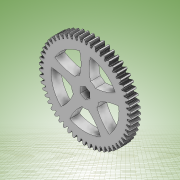
# Autodesk Inventor part: Engranaje1
Saved by Autodesk Inventor 2022 (Build 260153000, 153)
## iProperties
Created: 2022-03-08
Part Number: Engranaje1
Material: Genérico
Document SubType Name: Modeling
Designer: Marco
Density: 1 g/cm^3
Appearance: Valor por defecto
Author: Marco
Autodesk Inventor part; units mm, degrees
(part 1 of 3)
ref_plane "YZ Plane" through (0, 0, 0) normal (1, 0, 0) x (0, 1, 0)
ref_plane "XZ Plane" through (0, 0, 0) normal (0, 1, 0) x (-1, 0, 0)
ref_plane "XY Plane" through (0, 0, 0) normal (0, 0, 1) x (1, 0, 0)
sketch "Boceto4" plane through (0, 0, 0) normal (0, 0, 1) x (1, 0, 0)
  line L0 (-27.9789, -4.3637) -> (-27.7782, -4.2363)
  line L1 (-27.7782, -4.2363) -> (-27.5853, -4.1195)
  line L2 (-27.5853, -4.1195) -> (-27.3996, -4.0123)
  line L3 (-27.3996, -4.0123) -> (-27.2225, -3.9149)
  line L4 (-27.2225, -3.9149) -> (-27.053, -3.8263)
  line L5 (-27.053, -3.8263) -> (-26.8909, -3.7458)
  line L6 (-26.8909, -3.7458) -> (-26.7383, -3.674)
  line L7 (-26.7383, -3.674) -> (-26.5947, -3.6101)
  line L8 (-26.5947, -3.6101) -> (-26.3334, -3.5033)
  line L9 (-26.3334, -3.5033) -> (-26.0405, -3.3979)
  line L10 (-26.0405, -3.3979) -> (-25.9691, -3.3666)
  line L11 (-25.9691, -3.3666) -> (-25.9105, -3.334)
  line L12 (-25.9105, -3.334) -> (-25.8646, -3.3007)
  line L13 (-25.8646, -3.3007) -> (-25.8314, -3.2672)
  line L14 (-25.8314, -3.2672) -> (-25.811, -3.234)
  line L15 (-25.811, -3.234) -> (-25.8032, -3.2017)
  line L16 (-25.8032, -3.2017) -> (-25.8065, -3.1668)
  line L17 (-25.8065, -3.1668) -> (-25.8305, -2.9638)
  line L18 (-25.8305, -2.9638) -> (-25.8531, -2.7606)
  line L19 (-25.8531, -2.7606) -> (-25.8578, -2.7259)
  line L20 (-25.8578, -2.7259) -> (-25.8727, -2.6961)
  line L21 (-25.8727, -2.6961) -> (-25.9001, -2.6684)
  line L22 (-25.9001, -2.6684) -> (-25.94, -2.6433)
  line L23 (-25.94, -2.6433) -> (-25.9923, -2.6212)
  line L24 (-25.9923, -2.6212) -> (-26.0568, -2.6028)
  line L25 (-26.0568, -2.6028) -> (-26.1334, -2.5885)
  line L26 (-26.1334, -2.5885) -> (-26.4426, -2.5522)
  line L27 (-26.4426, -2.5522) -> (-26.7213, -2.5074)
  line L28 (-26.7213, -2.5074) -> (-26.8756, -2.4776)
  line L29 (-26.8756, -2.4776) -> (-27.0405, -2.4422)
  line L30 (-27.0405, -2.4422) -> (-27.2165, -2.4006)
  line L31 (-27.2165, -2.4006) -> (-27.4017, -2.3526)
  line L32 (-27.4017, -2.3526) -> (-27.5963, -2.2979)
  line L33 (-27.5963, -2.2979) -> (-27.8015, -2.2355)
  line L34 (-27.8015, -2.2355) -> (-28.0158, -2.1654)
  line L35 (-28.0158, -2.1654) -> (-28.2402, -2.0868)
  line L36 (-28.2402, -2.0868) -> (-28.4286, -2.0167)
  arc A0 (-28.4731, -1.2371) -> (-28.4286, -2.0167) centre (0, 0) ccw
  line L37 (-28.4731, -1.2371) -> (-28.294, -1.1459)
  line L38 (-28.294, -1.1459) -> (-28.0801, -1.0422)
  line L39 (-28.0801, -1.0422) -> (-27.8751, -0.9482)
  line L40 (-27.8751, -0.9482) -> (-27.6784, -0.8628)
  line L41 (-27.6784, -0.8628) -> (-27.4913, -0.7863)
  line L42 (-27.4913, -0.7863) -> (-27.3128, -0.7175)
  line L43 (-27.3128, -0.7175) -> (-27.1426, -0.6561)
  line L44 (-27.1426, -0.6561) -> (-26.9829, -0.6021)
  line L45 (-26.9829, -0.6021) -> (-26.8329, -0.555)
  line L46 (-26.8329, -0.555) -> (-26.5611, -0.4787)
  line L47 (-26.5611, -0.4787) -> (-26.2581, -0.4074)
  line L48 (-26.2581, -0.4074) -> (-26.1836, -0.3844)
  line L49 (-26.1836, -0.3844) -> (-26.1216, -0.3587)
  line L50 (-26.1216, -0.3587) -> (-26.0722, -0.3309)
  line L51 (-26.0722, -0.3309) -> (-26.0355, -0.3014)
  line L52 (-26.0355, -0.3014) -> (-26.0114, -0.2707)
  line L53 (-26.0114, -0.2707) -> (-26, -0.2394)
  line L54 (-26, -0.2394) -> (-25.9993, -0.2044)
  line L55 (-25.9993, -0.2044) -> (-26, 0)
  line L56 (-26, 0) -> (-25.9993, 0.2044)
  line L57 (-25.9993, 0.2044) -> (-26, 0.2394)
  line L58 (-26, 0.2394) -> (-26.0114, 0.2707)
  line L59 (-26.0114, 0.2707) -> (-26.0355, 0.3014)
  line L60 (-26.0355, 0.3014) -> (-26.0722, 0.3309)
  line L61 (-26.0722, 0.3309) -> (-26.1216, 0.3587)
  line L62 (-26.1216, 0.3587) -> (-26.1836, 0.3844)
  line L63 (-26.1836, 0.3844) -> (-26.2581, 0.4074)
  line L64 (-26.2581, 0.4074) -> (-26.5611, 0.4787)
  line L65 (-26.5611, 0.4787) -> (-26.8329, 0.555)
  line L66 (-26.8329, 0.555) -> (-26.9829, 0.6021)
  line L67 (-26.9829, 0.6021) -> (-27.1426, 0.6561)
  line L68 (-27.1426, 0.6561) -> (-27.3128, 0.7175)
  line L69 (-27.3128, 0.7175) -> (-27.4913, 0.7862)
  line L70 (-27.4913, 0.7862) -> (-27.6784, 0.8628)
  line L71 (-27.6784, 0.8628) -> (-27.8751, 0.9482)
  line L72 (-27.8751, 0.9482) -> (-28.0801, 1.0422)
  line L73 (-28.0801, 1.0422) -> (-28.294, 1.1459)
  line L74 (-28.294, 1.1459) -> (-28.4731, 1.2371)
  arc A1 (-28.4286, 2.0167) -> (-28.4731, 1.2371) centre (0, 0) ccw
  line L75 (-28.4286, 2.0167) -> (-28.2402, 2.0868)
  line L76 (-28.2402, 2.0868) -> (-28.0158, 2.1654)
  line L77 (-28.0158, 2.1654) -> (-27.8015, 2.2355)
  line L78 (-27.8015, 2.2355) -> (-27.5963, 2.2979)
  line L79 (-27.5963, 2.2979) -> (-27.4017, 2.3526)
  line L80 (-27.4017, 2.3526) -> (-27.2165, 2.4006)
  line L81 (-27.2165, 2.4006) -> (-27.0405, 2.4422)
  line L82 (-27.0405, 2.4422) -> (-26.8756, 2.4776)
  line L83 (-26.8756, 2.4776) -> (-26.7213, 2.5074)
  line L84 (-26.7213, 2.5074) -> (-26.4426, 2.5522)
  line L85 (-26.4426, 2.5522) -> (-26.1334, 2.5885)
  line L86 (-26.1334, 2.5885) -> (-26.0568, 2.6028)
  line L87 (-26.0568, 2.6028) -> (-25.9923, 2.6212)
  line L88 (-25.9923, 2.6212) -> (-25.94, 2.6433)
  line L89 (-25.94, 2.6433) -> (-25.9001, 2.6684)
  line L90 (-25.9001, 2.6684) -> (-25.8727, 2.6961)
  line L91 (-25.8727, 2.6961) -> (-25.8578, 2.7259)
  line L92 (-25.8578, 2.7259) -> (-25.8531, 2.7606)
  line L93 (-25.8531, 2.7606) -> (-25.8305, 2.9638)
  line L94 (-25.8305, 2.9638) -> (-25.8065, 3.1668)
  line L95 (-25.8065, 3.1668) -> (-25.8032, 3.2017)
  line L96 (-25.8032, 3.2017) -> (-25.811, 3.234)
  line L97 (-25.811, 3.234) -> (-25.8314, 3.2672)
  line L98 (-25.8314, 3.2672) -> (-25.8646, 3.3007)
  line L99 (-25.8646, 3.3007) -> (-25.9105, 3.334)
  line L100 (-25.9105, 3.334) -> (-25.9691, 3.3666)
  line L101 (-25.9691, 3.3666) -> (-26.0405, 3.3979)
  line L102 (-26.0405, 3.3979) -> (-26.3334, 3.5033)
  line L103 (-26.3334, 3.5033) -> (-26.5947, 3.6101)
  line L104 (-26.5947, 3.6101) -> (-26.7383, 3.674)
  line L105 (-26.7383, 3.674) -> (-26.8909, 3.7458)
  line L106 (-26.8909, 3.7458) -> (-27.053, 3.8263)
  line L107 (-27.053, 3.8263) -> (-27.2225, 3.9149)
  line L108 (-27.2225, 3.9149) -> (-27.3996, 4.0123)
  line L109 (-27.3996, 4.0123) -> (-27.5853, 4.1195)
  line L110 (-27.5853, 4.1195) -> (-27.7782, 4.2363)
  line L111 (-27.7782, 4.2363) -> (-27.9789, 4.3637)
  line L112 (-27.9789, 4.3637) -> (-28.1465, 4.4747)
  arc A2 (-28.0134, 5.2442) -> (-28.1465, 4.4747) centre (0, 0) ccw
  line L113 (-28.0134, 5.2442) -> (-27.8182, 5.2924)
  line L114 (-27.8182, 5.2924) -> (-27.5864, 5.3449)
  line L115 (-27.5864, 5.3449) -> (-27.3654, 5.3901)
  line L116 (-27.3654, 5.3901) -> (-27.1545, 5.4287)
  line L117 (-27.1545, 5.4287) -> (-26.9549, 5.4609)
  line L118 (-26.9549, 5.4609) -> (-26.7655, 5.4874)
  line L119 (-26.7655, 5.4874) -> (-26.5858, 5.5087)
  line L120 (-26.5858, 5.5087) -> (-26.418, 5.525)
  line L121 (-26.418, 5.525) -> (-26.2613, 5.537)
  line L122 (-26.2613, 5.537) -> (-25.9793, 5.5498)
  line L123 (-25.9793, 5.5498) -> (-25.668, 5.5506)
  line L124 (-25.668, 5.5506) -> (-25.5902, 5.5561)
  line L125 (-25.5902, 5.5561) -> (-25.524, 5.5671)
  line L126 (-25.524, 5.5671) -> (-25.4696, 5.583)
  line L127 (-25.4696, 5.583) -> (-25.4271, 5.6034)
  line L128 (-25.4271, 5.6034) -> (-25.3967, 5.6278)
  line L129 (-25.3967, 5.6278) -> (-25.3785, 5.6557)
  line L130 (-25.3785, 5.6557) -> (-25.3699, 5.6896)
  line L131 (-25.3699, 5.6896) -> (-25.3243, 5.8889)
  line L132 (-25.3243, 5.8889) -> (-25.2773, 6.0879)
  line L133 (-25.2773, 6.0879) -> (-25.2701, 6.1221)
  line L134 (-25.2701, 6.1221) -> (-25.2741, 6.1552)
  line L135 (-25.2741, 6.1552) -> (-25.2906, 6.1905)
  line L136 (-25.2906, 6.1905) -> (-25.3197, 6.2276)
  line L137 (-25.3197, 6.2276) -> (-25.3615, 6.2659)
  line L138 (-25.3615, 6.2659) -> (-25.4161, 6.3049)
  line L139 (-25.4161, 6.3049) -> (-25.4834, 6.3442)
  line L140 (-25.4834, 6.3442) -> (-25.7624, 6.4823)
  line L141 (-25.7624, 6.4823) -> (-26.0099, 6.6181)
  line L142 (-26.0099, 6.6181) -> (-26.1452, 6.698)
  line L143 (-26.1452, 6.698) -> (-26.2886, 6.7867)
  line L144 (-26.2886, 6.7867) -> (-26.4405, 6.8851)
  line L145 (-26.4405, 6.8851) -> (-26.5988, 6.9925)
  line L146 (-26.5988, 6.9925) -> (-26.7637, 7.1095)
  line L147 (-26.7637, 7.1095) -> (-26.9359, 7.2371)
  line L148 (-26.9359, 7.2371) -> (-27.1142, 7.3752)
  line L149 (-27.1142, 7.3752) -> (-27.2991, 7.5246)
  line L150 (-27.2991, 7.5246) -> (-27.453, 7.654)
  arc A3 (-27.233, 8.4033) -> (-27.453, 7.654) centre (0, 0) ccw
  line L151 (-27.233, 8.4033) -> (-27.0336, 8.4289)
  line L152 (-27.0336, 8.4289) -> (-26.7973, 8.4547)
  line L153 (-26.7973, 8.4547) -> (-26.5726, 8.4744)
  line L154 (-26.5726, 8.4744) -> (-26.3587, 8.4887)
  line L155 (-26.3587, 8.4887) -> (-26.1567, 8.4979)
  line L156 (-26.1567, 8.4979) -> (-25.9655, 8.5027)
  line L157 (-25.9655, 8.5027) -> (-25.7846, 8.5033)
  line L158 (-25.7846, 8.5033) -> (-25.616, 8.5005)
  line L159 (-25.616, 8.5005) -> (-25.4589, 8.4945)
  line L160 (-25.4589, 8.4945) -> (-25.1773, 8.475)
  line L161 (-25.1773, 8.475) -> (-24.868, 8.4403)
  line L162 (-24.868, 8.4403) -> (-24.7901, 8.4369)
  line L163 (-24.7901, 8.4369) -> (-24.7231, 8.4403)
  line L164 (-24.7231, 8.4403) -> (-24.6672, 8.4499)
  line L165 (-24.6672, 8.4499) -> (-24.6226, 8.4654)
  line L166 (-24.6226, 8.4654) -> (-24.5896, 8.4861)
  line L167 (-24.5896, 8.4861) -> (-24.5684, 8.5118)
  line L168 (-24.5684, 8.5118) -> (-24.556, 8.5445)
  line L169 (-24.556, 8.5445) -> (-24.488, 8.7373)
  line L170 (-24.488, 8.7373) -> (-24.4186, 8.9296)
  line L171 (-24.4186, 8.9296) -> (-24.4075, 8.9628)
  line L172 (-24.4075, 8.9628) -> (-24.4077, 8.9961)
  line L173 (-24.4077, 8.9961) -> (-24.4201, 9.033)
  line L174 (-24.4201, 9.033) -> (-24.4448, 9.0732)
  line L175 (-24.4448, 9.0732) -> (-24.482, 9.116)
  line L176 (-24.482, 9.116) -> (-24.5317, 9.161)
  line L177 (-24.5317, 9.161) -> (-24.5942, 9.2077)
  line L178 (-24.5942, 9.2077) -> (-24.8556, 9.3767)
  line L179 (-24.8556, 9.3767) -> (-25.0859, 9.5399)
  line L180 (-25.0859, 9.5399) -> (-25.2113, 9.6347)
  line L181 (-25.2113, 9.6347) -> (-25.3437, 9.7392)
  line L182 (-25.3437, 9.7392) -> (-25.4833, 9.8542)
  line L183 (-25.4833, 9.8542) -> (-25.6283, 9.979)
  line L184 (-25.6283, 9.979) -> (-25.7788, 10.1139)
  line L185 (-25.7788, 10.1139) -> (-25.9354, 10.2604)
  line L186 (-25.9354, 10.2604) -> (-26.0968, 10.4179)
  line L187 (-26.0968, 10.4179) -> (-26.2634, 10.5874)
  line L188 (-26.2634, 10.5874) -> (-26.4016, 10.7335)
  arc A4 (-26.0976, 11.4528) -> (-26.4016, 10.7335) centre (0, 0) ccw
  line L189 (-26.0976, 11.4528) -> (-25.8966, 11.4556)
  line L190 (-25.8966, 11.4556) -> (-25.6588, 11.4542)
  line L191 (-25.6588, 11.4542) -> (-25.4334, 11.4482)
  line L192 (-25.4334, 11.4482) -> (-25.2192, 11.438)
  line L193 (-25.2192, 11.438) -> (-25.0175, 11.4242)
  line L194 (-25.0175, 11.4242) -> (-24.827, 11.4071)
  line L195 (-24.827, 11.4071) -> (-24.6472, 11.3871)
  line L196 (-24.6472, 11.3871) -> (-24.4801, 11.3651)
  line L197 (-24.4801, 11.3651) -> (-24.3247, 11.3412)
  line L198 (-24.3247, 11.3412) -> (-24.0471, 11.2898)
  line L199 (-24.0471, 11.2898) -> (-23.7437, 11.22)
  line L200 (-23.7437, 11.22) -> (-23.6668, 11.2078)
  line L201 (-23.6668, 11.2078) -> (-23.5998, 11.2035)
  line L202 (-23.5998, 11.2035) -> (-23.5432, 11.2067)
  line L203 (-23.5432, 11.2067) -> (-23.4972, 11.2169)
  line L204 (-23.4972, 11.2169) -> (-23.462, 11.2338)
  line L205 (-23.462, 11.2338) -> (-23.438, 11.2569)
  line L206 (-23.438, 11.2569) -> (-23.4219, 11.288)
  line L207 (-23.4219, 11.288) -> (-23.3324, 11.4717)
  line L208 (-23.3324, 11.4717) -> (-23.2415, 11.6549)
  line L209 (-23.2415, 11.6549) -> (-23.2267, 11.6866)
  line L210 (-23.2267, 11.6866) -> (-23.2231, 11.7197)
  line L211 (-23.2231, 11.7197) -> (-23.2312, 11.7578)
  line L212 (-23.2312, 11.7578) -> (-23.2512, 11.8005)
  line L213 (-23.2512, 11.8005) -> (-23.2832, 11.8473)
  line L214 (-23.2832, 11.8473) -> (-23.3275, 11.8977)
  line L215 (-23.3275, 11.8977) -> (-23.3842, 11.9512)
  line L216 (-23.3842, 11.9512) -> (-23.6247, 12.1489)
  line L217 (-23.6247, 12.1489) -> (-23.8349, 12.3373)
  line L218 (-23.8349, 12.3373) -> (-23.9487, 12.4458)
  line L219 (-23.9487, 12.4458) -> (-24.0683, 12.5647)
  line L220 (-24.0683, 12.5647) -> (-24.1939, 12.6949)
  line L221 (-24.1939, 12.6949) -> (-24.3237, 12.8353)
  line L222 (-24.3237, 12.8353) -> (-24.4579, 12.9866)
  line L223 (-24.4579, 12.9866) -> (-24.5967, 13.15)
  line L224 (-24.5967, 13.15) -> (-24.7391, 13.3248)
  line L225 (-24.7391, 13.3248) -> (-24.8854, 13.5122)
  line L226 (-24.8854, 13.5122) -> (-25.0059, 13.6731)
  arc A5 (-24.6219, 14.3531) -> (-25.0059, 13.6731) centre (0, 0) ccw
  line L227 (-24.6219, 14.3531) -> (-24.4219, 14.3329)
  line L228 (-24.4219, 14.3329) -> (-24.1859, 14.3044)
  line L229 (-24.1859, 14.3044) -> (-23.9626, 14.2728)
  line L230 (-23.9626, 14.2728) -> (-23.751, 14.2382)
  line L231 (-23.751, 14.2382) -> (-23.5522, 14.2015)
  line L232 (-23.5522, 14.2015) -> (-23.3649, 14.1628)
  line L233 (-23.3649, 14.1628) -> (-23.1885, 14.1225)
  line L234 (-23.1885, 14.1225) -> (-23.025, 14.0815)
  line L235 (-23.025, 14.0815) -> (-22.8733, 14.0401)
  line L236 (-22.8733, 14.0401) -> (-22.6034, 13.9573)
  line L237 (-22.6034, 13.9573) -> (-22.31, 13.8535)
  line L238 (-22.31, 13.8535) -> (-22.2349, 13.8325)
  line L239 (-22.2349, 13.8325) -> (-22.1689, 13.8206)
  line L240 (-22.1689, 13.8206) -> (-22.1122, 13.8174)
  line L241 (-22.1122, 13.8174) -> (-22.0654, 13.8223)
  line L242 (-22.0654, 13.8223) -> (-22.0285, 13.8351)
  line L243 (-22.0285, 13.8351) -> (-22.002, 13.8552)
  line L244 (-22.002, 13.8552) -> (-21.9825, 13.8843)
  line L245 (-21.9825, 13.8843) -> (-21.8726, 14.0567)
  line L246 (-21.8726, 14.0567) -> (-21.7615, 14.2282)
  line L247 (-21.7615, 14.2282) -> (-21.7431, 14.2581)
  line L248 (-21.7431, 14.2581) -> (-21.7358, 14.2906)
  line L249 (-21.7358, 14.2906) -> (-21.7395, 14.3294)
  line L250 (-21.7395, 14.3294) -> (-21.7545, 14.3741)
  line L251 (-21.7545, 14.3741) -> (-21.781, 14.4242)
  line L252 (-21.781, 14.4242) -> (-21.8192, 14.4793)
  line L253 (-21.8192, 14.4793) -> (-21.8695, 14.5389)
  line L254 (-21.8695, 14.5389) -> (-22.0858, 14.7627)
  line L255 (-22.0858, 14.7627) -> (-22.2732, 14.9738)
  line L256 (-22.2732, 14.9738) -> (-22.3739, 15.0946)
  line L257 (-22.3739, 15.0946) -> (-22.4791, 15.2263)
  line L258 (-22.4791, 15.2263) -> (-22.5891, 15.37)
  line L259 (-22.5891, 15.37) -> (-22.7021, 15.5243)
  line L260 (-22.7021, 15.5243) -> (-22.8181, 15.6899)
  line L261 (-22.8181, 15.6899) -> (-22.9374, 15.8681)
  line L262 (-22.9374, 15.8681) -> (-23.059, 16.058)
  line L263 (-23.059, 16.058) -> (-23.1829, 16.2609)
  line L264 (-23.1829, 16.2609) -> (-23.2843, 16.4344)
  arc A6 (-22.8253, 17.0662) -> (-23.2843, 16.4344) centre (0, 0) ccw
  line L265 (-22.8253, 17.0662) -> (-22.6289, 17.0233)
  line L266 (-22.6289, 17.0233) -> (-22.3977, 16.9682)
  line L267 (-22.3977, 16.9682) -> (-22.1795, 16.9113)
  line L268 (-22.1795, 16.9113) -> (-21.9732, 16.8528)
  line L269 (-21.9732, 16.8528) -> (-21.7799, 16.7937)
  line L270 (-21.7799, 16.7937) -> (-21.5982, 16.7339)
  line L271 (-21.5982, 16.7339) -> (-21.4275, 16.6737)
  line L272 (-21.4275, 16.6737) -> (-21.2697, 16.6144)
  line L273 (-21.2697, 16.6144) -> (-21.1238, 16.5559)
  line L274 (-21.1238, 16.5559) -> (-20.8651, 16.443)
  line L275 (-20.8651, 16.443) -> (-20.5854, 16.3063)
  line L276 (-20.5854, 16.3063) -> (-20.5132, 16.277)
  line L277 (-20.5132, 16.277) -> (-20.4489, 16.2576)
  line L278 (-20.4489, 16.2576) -> (-20.393, 16.2479)
  line L279 (-20.393, 16.2479) -> (-20.3459, 16.2475)
  line L280 (-20.3459, 16.2475) -> (-20.3079, 16.2559)
  line L281 (-20.3079, 16.2559) -> (-20.2793, 16.273)
  line L282 (-20.2793, 16.273) -> (-20.2565, 16.2996)
  line L283 (-20.2565, 16.2996) -> (-20.1277, 16.4583)
  line L284 (-20.1277, 16.4583) -> (-19.9977, 16.6161)
  line L285 (-19.9977, 16.6161) -> (-19.9761, 16.6437)
  line L286 (-19.9761, 16.6437) -> (-19.9651, 16.6751)
  line L287 (-19.9651, 16.6751) -> (-19.9644, 16.7141)
  line L288 (-19.9644, 16.7141) -> (-19.9741, 16.7602)
  line L289 (-19.9741, 16.7602) -> (-19.9948, 16.813)
  line L290 (-19.9948, 16.813) -> (-20.0265, 16.8721)
  line L291 (-20.0265, 16.8721) -> (-20.0696, 16.9371)
  line L292 (-20.0696, 16.9371) -> (-20.2591, 17.1841)
  line L293 (-20.2591, 17.1841) -> (-20.4212, 17.4152)
  line L294 (-20.4212, 17.4152) -> (-20.5074, 17.5466)
  line L295 (-20.5074, 17.5466) -> (-20.5969, 17.6895)
  line L296 (-20.5969, 17.6895) -> (-20.6898, 17.8448)
  line L297 (-20.6898, 17.8448) -> (-20.7844, 18.011)
  line L298 (-20.7844, 18.011) -> (-20.8808, 18.1887)
  line L299 (-20.8808, 18.1887) -> (-20.9791, 18.3793)
  line L300 (-20.9791, 18.3793) -> (-21.0782, 18.5819)
  line L301 (-21.0782, 18.5819) -> (-21.1782, 18.7975)
  line L302 (-21.1782, 18.7975) -> (-21.2592, 18.9815)
  arc A7 (-20.7311, 19.5568) -> (-21.2592, 18.9815) centre (0, 0) ccw
  line L303 (-20.7311, 19.5568) -> (-20.5409, 19.4919)
  line L304 (-20.5409, 19.4919) -> (-20.3175, 19.4107)
  line L305 (-20.3175, 19.4107) -> (-20.1072, 19.3293)
  line L306 (-20.1072, 19.3293) -> (-19.9089, 19.2477)
  line L307 (-19.9089, 19.2477) -> (-19.7236, 19.1669)
  line L308 (-19.7236, 19.1669) -> (-19.5499, 19.0868)
  line L309 (-19.5499, 19.0868) -> (-19.3872, 19.0076)
  line L310 (-19.3872, 19.0076) -> (-19.2372, 18.9306)
  line L311 (-19.2372, 18.9306) -> (-19.0988, 18.856)
  line L312 (-19.0988, 18.856) -> (-18.8547, 18.7142)
  line L313 (-18.8547, 18.7142) -> (-18.5924, 18.5466)
  line L314 (-18.5924, 18.5466) -> (-18.524, 18.5092)
  line L315 (-18.524, 18.5092) -> (-18.4624, 18.4826)
  line L316 (-18.4624, 18.4826) -> (-18.408, 18.4666)
  line L317 (-18.408, 18.4666) -> (-18.3612, 18.4608)
  line L318 (-18.3612, 18.4608) -> (-18.3224, 18.4649)
  line L319 (-18.3224, 18.4649) -> (-18.2921, 18.4786)
  line L320 (-18.2921, 18.4786) -> (-18.2665, 18.5024)
  line L321 (-18.2665, 18.5024) -> (-18.1204, 18.6454)
  line L322 (-18.1204, 18.6454) -> (-17.9733, 18.7874)
  line L323 (-17.9733, 18.7874) -> (-17.9487, 18.8123)
  line L324 (-17.9487, 18.8123) -> (-17.9342, 18.8423)
  line L325 (-17.9342, 18.8423) -> (-17.929, 18.8809)
  line L326 (-17.929, 18.8809) -> (-17.9334, 18.9278)
  line L327 (-17.9334, 18.9278) -> (-17.9479, 18.9827)
  line L328 (-17.9479, 18.9827) -> (-17.9727, 19.045)
  line L329 (-17.9727, 19.045) -> (-18.0081, 19.1145)
  line L330 (-18.0081, 19.1145) -> (-18.1682, 19.3814)
  line L331 (-18.1682, 19.3814) -> (-18.3029, 19.6295)
  line L332 (-18.3029, 19.6295) -> (-18.3736, 19.7699)
  line L333 (-18.3736, 19.7699) -> (-18.4462, 19.9221)
  line L334 (-18.4462, 19.9221) -> (-18.5207, 20.0869)
  line L335 (-18.5207, 20.0869) -> (-18.5959, 20.2628)
  line L336 (-18.5959, 20.2628) -> (-18.6714, 20.4504)
  line L337 (-18.6714, 20.4504) -> (-18.7473, 20.6509)
  line L338 (-18.7473, 20.6509) -> (-18.8226, 20.8635)
  line L339 (-18.8226, 20.8635) -> (-18.8974, 21.0891)
  line L340 (-18.8974, 21.0891) -> (-18.9569, 21.2812)
  arc A8 (-18.3667, 21.7925) -> (-18.9569, 21.2812) centre (0, 0) ccw
  line L341 (-18.3667, 21.7925) -> (-18.1851, 21.7063)
  line L342 (-18.1851, 21.7063) -> (-17.9724, 21.6002)
  line L343 (-17.9724, 21.6002) -> (-17.7727, 21.4954)
  line L344 (-17.7727, 21.4954) -> (-17.585, 21.3917)
  line L345 (-17.585, 21.3917) -> (-17.4101, 21.2903)
  line L346 (-17.4101, 21.2903) -> (-17.2467, 21.1909)
  line L347 (-17.2467, 21.1909) -> (-17.0941, 21.0937)
  line L348 (-17.0941, 21.0937) -> (-16.9539, 21.0001)
  line L349 (-16.9539, 21.0001) -> (-16.8249, 20.9102)
  line L350 (-16.8249, 20.9102) -> (-16.5986, 20.7415)
  line L351 (-16.5986, 20.7415) -> (-16.3571, 20.5451)
  line L352 (-16.3571, 20.5451) -> (-16.2934, 20.5001)
  line L353 (-16.2934, 20.5001) -> (-16.2352, 20.4667)
  line L354 (-16.2352, 20.4667) -> (-16.183, 20.4446)
  line L355 (-16.183, 20.4446) -> (-16.1372, 20.4335)
  line L356 (-16.1372, 20.4335) -> (-16.0982, 20.4331)
  line L357 (-16.0982, 20.4331) -> (-16.0665, 20.4432)
  line L358 (-16.0665, 20.4432) -> (-16.0383, 20.4641)
  line L359 (-16.0383, 20.4641) -> (-15.8768, 20.5895)
  line L360 (-15.8768, 20.5895) -> (-15.7145, 20.7137)
  line L361 (-15.7145, 20.7137) -> (-15.6872, 20.7357)
  line L362 (-15.6872, 20.7357) -> (-15.6694, 20.7638)
  line L363 (-15.6694, 20.7638) -> (-15.6598, 20.8016)
  line L364 (-15.6598, 20.8016) -> (-15.6589, 20.8487)
  line L365 (-15.6589, 20.8487) -> (-15.667, 20.9048)
  line L366 (-15.667, 20.9048) -> (-15.6846, 20.9696)
  line L367 (-15.6846, 20.9696) -> (-15.7118, 21.0426)
  line L368 (-15.7118, 21.0426) -> (-15.8404, 21.3261)
  line L369 (-15.8404, 21.3261) -> (-15.946, 21.5879)
  line L370 (-15.946, 21.5879) -> (-16.0002, 21.7355)
  line L371 (-16.0002, 21.7355) -> (-16.055, 21.8949)
  line L372 (-16.055, 21.8949) -> (-16.1103, 22.0672)
  line L373 (-16.1103, 22.0672) -> (-16.1649, 22.2505)
  line L374 (-16.1649, 22.2505) -> (-16.2185, 22.4455)
  line L375 (-16.2185, 22.4455) -> (-16.271, 22.6533)
  line L376 (-16.271, 22.6533) -> (-16.3217, 22.8731)
  line L377 (-16.3217, 22.8731) -> (-16.3702, 23.1058)
  line L378 (-16.3702, 23.1058) -> (-16.4074, 23.3034)
  arc A9 (-15.7628, 23.7441) -> (-16.4074, 23.3034) centre (0, 0) ccw
  line L379 (-15.7628, 23.7441) -> (-15.5922, 23.6378)
  line L380 (-15.5922, 23.6378) -> (-15.393, 23.5081)
  line L381 (-15.393, 23.5081) -> (-15.2066, 23.3812)
  line L382 (-15.2066, 23.3812) -> (-15.0319, 23.2568)
  line L383 (-15.0319, 23.2568) -> (-14.8697, 23.1361)
  line L384 (-14.8697, 23.1361) -> (-14.7187, 23.0187)
  line L385 (-14.7187, 23.0187) -> (-14.5782, 22.9048)
  line L386 (-14.5782, 22.9048) -> (-14.4495, 22.7958)
  line L387 (-14.4495, 22.7958) -> (-14.3317, 22.6917)
  line L388 (-14.3317, 22.6917) -> (-14.126, 22.4984)
  line L389 (-14.126, 22.4984) -> (-13.9085, 22.2757)
  line L390 (-13.9085, 22.2757) -> (-13.8503, 22.2238)
  line L391 (-13.8503, 22.2238) -> (-13.7963, 22.184)
  line L392 (-13.7963, 22.184) -> (-13.747, 22.1561)
  line L393 (-13.747, 22.1561) -> (-13.7027, 22.1398)
  line L394 (-13.7027, 22.1398) -> (-13.664, 22.135)
  line L395 (-13.664, 22.135) -> (-13.6314, 22.1414)
  line L396 (-13.6314, 22.1414) -> (-13.601, 22.1589)
  line L397 (-13.601, 22.1589) -> (-13.4263, 22.2651)
  line L398 (-13.4263, 22.2651) -> (-13.2509, 22.37)
  line L399 (-13.2509, 22.37) -> (-13.2213, 22.3887)
  line L400 (-13.2213, 22.3887) -> (-13.2004, 22.4146)
  line L401 (-13.2004, 22.4146) -> (-13.1866, 22.4511)
  line L402 (-13.1866, 22.4511) -> (-13.1803, 22.4978)
  line L403 (-13.1803, 22.4978) -> (-13.1819, 22.5545)
  line L404 (-13.1819, 22.5545) -> (-13.192, 22.6208)
  line L405 (-13.192, 22.6208) -> (-13.2108, 22.6965)
  line L406 (-13.2108, 22.6965) -> (-13.3062, 22.9928)
  line L407 (-13.3062, 22.9928) -> (-13.3812, 23.2649)
  line L408 (-13.3812, 23.2649) -> (-13.4182, 23.4177)
  line L409 (-13.4182, 23.4177) -> (-13.4546, 23.5824)
  line L410 (-13.4546, 23.5824) -> (-13.4898, 23.7598)
  line L411 (-13.4898, 23.7598) -> (-13.5231, 23.9482)
  line L412 (-13.5231, 23.9482) -> (-13.5542, 24.1479)
  line L413 (-13.5542, 24.1479) -> (-13.5827, 24.3604)
  line L414 (-13.5827, 24.3604) -> (-13.608, 24.5845)
  line L415 (-13.608, 24.5845) -> (-13.6296, 24.8213)
  line L416 (-13.6296, 24.8213) -> (-13.6441, 25.0218)
  arc A10 (-12.9534, 25.3862) -> (-13.6441, 25.0218) centre (0, 0) ccw
  line L417 (-12.9534, 25.3862) -> (-12.7961, 25.2611)
  line L418 (-12.7961, 25.2611) -> (-12.6129, 25.1096)
  line L419 (-12.6129, 25.1096) -> (-12.4422, 24.9622)
  line L420 (-12.4422, 24.9622) -> (-12.2829, 24.8187)
  line L421 (-12.2829, 24.8187) -> (-12.1355, 24.6803)
  line L422 (-12.1355, 24.6803) -> (-11.9988, 24.5465)
  line L423 (-11.9988, 24.5465) -> (-11.8722, 24.4173)
  line L424 (-11.8722, 24.4173) -> (-11.7568, 24.2943)
  line L425 (-11.7568, 24.2943) -> (-11.6516, 24.1775)
  line L426 (-11.6516, 24.1775) -> (-11.4693, 23.962)
  line L427 (-11.4693, 23.962) -> (-11.2786, 23.716)
  line L428 (-11.2786, 23.716) -> (-11.2267, 23.6578)
  line L429 (-11.2267, 23.6578) -> (-11.1776, 23.6121)
  line L430 (-11.1776, 23.6121) -> (-11.1318, 23.5787)
  line L431 (-11.1318, 23.5787) -> (-11.0897, 23.5575)
  line L432 (-11.0897, 23.5575) -> (-11.0518, 23.5483)
  line L433 (-11.0518, 23.5483) -> (-11.0186, 23.551)
  line L434 (-11.0186, 23.551) -> (-10.9864, 23.5649)
  line L435 (-10.9864, 23.5649) -> (-10.8008, 23.6504)
  line L436 (-10.8008, 23.6504) -> (-10.6145, 23.7347)
  line L437 (-10.6145, 23.7347) -> (-10.583, 23.7499)
  line L438 (-10.583, 23.7499) -> (-10.5593, 23.7732)
  line L439 (-10.5593, 23.7732) -> (-10.5414, 23.8079)
  line L440 (-10.5414, 23.8079) -> (-10.5298, 23.8536)
  line L441 (-10.5298, 23.8536) -> (-10.525, 23.9101)
  line L442 (-10.525, 23.9101) -> (-10.5274, 23.9771)
  line L443 (-10.5274, 23.9771) -> (-10.5374, 24.0545)
  line L444 (-10.5374, 24.0545) -> (-10.5985, 24.3597)
  line L445 (-10.5985, 24.3597) -> (-10.642, 24.6386)
  line L446 (-10.642, 24.6386) -> (-10.6614, 24.7946)
  line L447 (-10.6614, 24.7946) -> (-10.6787, 24.9623)
  line L448 (-10.6787, 24.9623) -> (-10.6935, 25.1426)
  line L449 (-10.6935, 25.1426) -> (-10.7051, 25.3336)
  line L450 (-10.7051, 25.3336) -> (-10.7132, 25.5356)
  line L451 (-10.7132, 25.5356) -> (-10.7173, 25.75)
  line L452 (-10.7173, 25.75) -> (-10.7168, 25.9755)
  line L453 (-10.7168, 25.9755) -> (-10.7114, 26.2131)
  line L454 (-10.7114, 26.2131) -> (-10.7029, 26.414)
  arc A11 (-9.9752, 26.6973) -> (-10.7029, 26.414) centre (0, 0) ccw
  line L455 (-9.9752, 26.6973) -> (-9.8331, 26.5551)
  line L456 (-9.8331, 26.5551) -> (-9.6684, 26.3836)
  line L457 (-9.6684, 26.3836) -> (-9.5156, 26.2178)
  line L458 (-9.5156, 26.2178) -> (-9.3737, 26.0571)
  line L459 (-9.3737, 26.0571) -> (-9.243, 25.9028)
  line L460 (-9.243, 25.9028) -> (-9.1225, 25.7543)
  line L461 (-9.1225, 25.7543) -> (-9.0115, 25.6114)
  line L462 (-9.0115, 25.6114) -> (-8.9108, 25.4762)
  line L463 (-8.9108, 25.4762) -> (-8.8196, 25.3481)
  line L464 (-8.8196, 25.3481) -> (-8.6631, 25.1132)
  line L465 (-8.6631, 25.1132) -> (-8.5017, 24.8471)
  line L466 (-8.5017, 24.8471) -> (-8.4568, 24.7833)
  line L467 (-8.4568, 24.7833) -> (-8.4132, 24.7323)
  line L468 (-8.4132, 24.7323) -> (-8.3714, 24.6939)
  line L469 (-8.3714, 24.6939) -> (-8.332, 24.6681)
  line L470 (-8.332, 24.6681) -> (-8.2954, 24.6546)
  line L471 (-8.2954, 24.6546) -> (-8.2622, 24.6535)
  line L472 (-8.2622, 24.6535) -> (-8.2286, 24.6636)
  line L473 (-8.2286, 24.6636) -> (-8.0344, 24.7275)
  line L474 (-8.0344, 24.7275) -> (-7.8398, 24.79)
  line L475 (-7.8398, 24.79) -> (-7.8067, 24.8015)
  line L476 (-7.8067, 24.8015) -> (-7.7805, 24.8219)
  line L477 (-7.7805, 24.8219) -> (-7.7588, 24.8543)
  line L478 (-7.7588, 24.8543) -> (-7.7421, 24.8984)
  line L479 (-7.7421, 24.8984) -> (-7.7309, 24.954)
  line L480 (-7.7309, 24.954) -> (-7.7256, 25.0209)
  line L481 (-7.7256, 25.0209) -> (-7.7268, 25.0988)
  line L482 (-7.7268, 25.0988) -> (-7.7526, 25.4091)
  line L483 (-7.7526, 25.4091) -> (-7.764, 25.6911)
  line L484 (-7.764, 25.6911) -> (-7.7655, 25.8483)
  line L485 (-7.7655, 25.8483) -> (-7.7636, 26.0169)
  line L486 (-7.7636, 26.0169) -> (-7.7577, 26.1977)
  line L487 (-7.7577, 26.1977) -> (-7.7475, 26.3887)
  line L488 (-7.7475, 26.3887) -> (-7.7325, 26.5903)
  line L489 (-7.7325, 26.5903) -> (-7.7121, 26.8038)
  line L490 (-7.7121, 26.8038) -> (-7.686, 27.0278)
  line L491 (-7.686, 27.0278) -> (-7.6535, 27.2633)
  line L492 (-7.6535, 27.2633) -> (-7.6222, 27.4618)
  arc A12 (-6.8669, 27.6604) -> (-7.6222, 27.4618) centre (0, 0) ccw
  line L493 (-6.8669, 27.6604) -> (-6.742, 27.5029)
  line L494 (-6.742, 27.5029) -> (-6.5979, 27.3138)
  line L495 (-6.5979, 27.3138) -> (-6.465, 27.1316)
  line L496 (-6.465, 27.1316) -> (-6.3423, 26.9558)
  line L497 (-6.3423, 26.9558) -> (-6.2301, 26.7876)
  line L498 (-6.2301, 26.7876) -> (-6.1273, 26.6263)
  line L499 (-6.1273, 26.6263) -> (-6.0333, 26.4717)
  line L500 (-6.0333, 26.4717) -> (-5.9487, 26.3259)
  line L501 (-5.9487, 26.3259) -> (-5.8727, 26.1882)
  line L502 (-5.8727, 26.1882) -> (-5.7439, 25.937)
  line L503 (-5.7439, 25.937) -> (-5.6139, 25.6542)
  line L504 (-5.6139, 25.6542) -> (-5.5766, 25.5858)
  line L505 (-5.5766, 25.5858) -> (-5.5391, 25.5301)
  line L506 (-5.5391, 25.5301) -> (-5.502, 25.4872)
  line L507 (-5.502, 25.4872) -> (-5.4658, 25.4571)
  line L508 (-5.4658, 25.4571) -> (-5.4309, 25.4395)
  line L509 (-5.4309, 25.4395) -> (-5.398, 25.4346)
  line L510 (-5.398, 25.4346) -> (-5.3636, 25.4408)
  line L511 (-5.3636, 25.4408) -> (-5.1634, 25.4821)
  line L512 (-5.1634, 25.4821) -> (-4.9629, 25.522)
  line L513 (-4.9629, 25.522) -> (-4.9287, 25.5297)
  line L514 (-4.9287, 25.5297) -> (-4.9003, 25.5471)
  line L515 (-4.9003, 25.5471) -> (-4.875, 25.5768)
  line L516 (-4.875, 25.5768) -> (-4.8534, 25.6186)
  line L517 (-4.8534, 25.6186) -> (-4.8359, 25.6726)
  line L518 (-4.8359, 25.6726) -> (-4.8231, 25.7385)
  line L519 (-4.8231, 25.7385) -> (-4.8153, 25.816)
  line L520 (-4.8153, 25.816) -> (-4.8056, 26.1272)
  line L521 (-4.8056, 26.1272) -> (-4.7849, 26.4087)
  line L522 (-4.7849, 26.4087) -> (-4.7684, 26.565)
  line L523 (-4.7684, 26.565) -> (-4.7473, 26.7323)
  line L524 (-4.7473, 26.7323) -> (-4.7208, 26.9113)
  line L525 (-4.7208, 26.9113) -> (-4.6889, 27.0999)
  line L526 (-4.6889, 27.0999) -> (-4.651, 27.2985)
  line L527 (-4.651, 27.2985) -> (-4.6065, 27.5082)
  line L528 (-4.6065, 27.5082) -> (-4.555, 27.7277)
  line L529 (-4.555, 27.7277) -> (-4.4958, 27.958)
  line L530 (-4.4958, 27.958) -> (-4.4421, 28.1517)
  arc A13 (-3.6691, 28.2628) -> (-4.4421, 28.1517) centre (0, 0) ccw
  line L531 (-3.6691, 28.2628) -> (-3.563, 28.0921)
  line L532 (-3.563, 28.0921) -> (-3.4414, 27.8879)
  line L533 (-3.4414, 27.8879) -> (-3.3301, 27.6917)
  line L534 (-3.3301, 27.6917) -> (-3.2282, 27.503)
  line L535 (-3.2282, 27.503) -> (-3.1359, 27.3232)
  line L536 (-3.1359, 27.3232) -> (-3.0522, 27.1512)
  line L537 (-3.0522, 27.1512) -> (-2.9764, 26.9869)
  line L538 (-2.9764, 26.9869) -> (-2.909, 26.8324)
  line L539 (-2.909, 26.8324) -> (-2.8492, 26.687)
  line L540 (-2.8492, 26.687) -> (-2.7499, 26.4227)
  line L541 (-2.7499, 26.4227) -> (-2.6529, 26.1269)
  line L542 (-2.6529, 26.1269) -> (-2.6237, 26.0547)
  line L543 (-2.6237, 26.0547) -> (-2.5928, 25.9951)
  line L544 (-2.5928, 25.9951) -> (-2.5608, 25.9483)
  line L545 (-2.5608, 25.9483) -> (-2.5282, 25.9142)
  line L546 (-2.5282, 25.9142) -> (-2.4957, 25.8928)
  line L547 (-2.4957, 25.8928) -> (-2.4635, 25.8841)
  line L548 (-2.4635, 25.8841) -> (-2.4286, 25.8864)
  line L549 (-2.4286, 25.8864) -> (-2.225, 25.9046)
  line L550 (-2.225, 25.9046) -> (-2.0212, 25.9214)
  line L551 (-2.0212, 25.9214) -> (-1.9864, 25.9251)
  line L552 (-1.9864, 25.9251) -> (-1.9562, 25.9391)
  line L553 (-1.9562, 25.9391) -> (-1.9277, 25.9657)
  line L554 (-1.9277, 25.9657) -> (-1.9015, 26.0049)
  line L555 (-1.9015, 26.0049) -> (-1.8779, 26.0565)
  line L556 (-1.8779, 26.0565) -> (-1.8577, 26.1205)
  line L557 (-1.8577, 26.1205) -> (-1.8411, 26.1967)
  line L558 (-1.8411, 26.1967) -> (-1.796, 26.5047)
  line L559 (-1.796, 26.5047) -> (-1.7433, 26.782)
  line L560 (-1.7433, 26.782) -> (-1.7091, 26.9354)
  line L561 (-1.7091, 26.9354) -> (-1.6691, 27.0992)
  line L562 (-1.6691, 27.0992) -> (-1.6224, 27.274)
  line L563 (-1.6224, 27.274) -> (-1.5692, 27.4577)
  line L564 (-1.5692, 27.4577) -> (-1.5089, 27.6507)
  line L565 (-1.5089, 27.6507) -> (-1.4407, 27.854)
  line L566 (-1.4407, 27.854) -> (-1.3645, 28.0662)
  line L567 (-1.3645, 28.0662) -> (-1.2795, 28.2882)
  line L568 (-1.2795, 28.2882) -> (-1.2041, 28.4746)
  arc A14 (-0.4235, 28.4969) -> (-1.2041, 28.4746) centre (0, 0) ccw
  line L569 (-0.4235, 28.4969) -> (-0.3375, 28.3151)
  line L570 (-0.3375, 28.3151) -> (-0.2399, 28.0984)
  line L571 (-0.2399, 28.0984) -> (-0.1518, 27.8908)
  line L572 (-0.1518, 27.8908) -> (-0.0721, 27.6917)
  line L573 (-0.0721, 27.6917) -> (-0.0009, 27.5025)
  line L574 (-0.0009, 27.5025) -> (0.0627, 27.3221)
  line L575 (0.0627, 27.3221) -> (0.1193, 27.1503)
  line L576 (0.1193, 27.1503) -> (0.1686, 26.9891)
  line L577 (0.1686, 26.9891) -> (0.2115, 26.8378)
  line L578 (0.2115, 26.8378) -> (0.28, 26.564)
  line L579 (0.28, 26.564) -> (0.3426, 26.259)
  line L580 (0.3426, 26.259) -> (0.3634, 26.1839)
  line L581 (0.3634, 26.1839) -> (0.3873, 26.1212)
  line L582 (0.3873, 26.1212) -> (0.4138, 26.071)
  line L583 (0.4138, 26.071) -> (0.4422, 26.0335)
  line L584 (0.4422, 26.0335) -> (0.4722, 26.0085)
  line L585 (0.4722, 26.0085) -> (0.5031, 25.9962)
  line L586 (0.5031, 25.9962) -> (0.5381, 25.9945)
  line L587 (0.5381, 25.9945) -> (0.7425, 25.9894)
  line L588 (0.7425, 25.9894) -> (0.9468, 25.9828)
  line L589 (0.9468, 25.9828) -> (0.9818, 25.9826)
  line L590 (0.9818, 25.9826) -> (1.0134, 25.993)
  line L591 (1.0134, 25.993) -> (1.0447, 26.0162)
  line L592 (1.0447, 26.0162) -> (1.0753, 26.0521)
  line L593 (1.0753, 26.0521) -> (1.1045, 26.1007)
  line L594 (1.1045, 26.1007) -> (1.132, 26.162)
  line L595 (1.132, 26.162) -> (1.1571, 26.2358)
  line L596 (1.1571, 26.2358) -> (1.237, 26.5366)
  line L597 (1.237, 26.5366) -> (1.321, 26.8061)
  line L598 (1.321, 26.8061) -> (1.3724, 26.9547)
  line L599 (1.3724, 26.9547) -> (1.4309, 27.1128)
  line L600 (1.4309, 27.1128) -> (1.4972, 27.2812)
  line L601 (1.4972, 27.2812) -> (1.571, 27.4576)
  line L602 (1.571, 27.4576) -> (1.6529, 27.6425)
  line L603 (1.6529, 27.6425) -> (1.7438, 27.8367)
  line L604 (1.7438, 27.8367) -> (1.8437, 28.0388)
  line L605 (1.8437, 28.0388) -> (1.9534, 28.2497)
  line L606 (1.9534, 28.2497) -> (2.0496, 28.4262)
  arc A15 (2.8277, 28.3594) -> (2.0496, 28.4262) centre (0, 0) ccw
  line L607 (2.8277, 28.3594) -> (2.8924, 28.1691)
  line L608 (2.8924, 28.1691) -> (2.9646, 27.9426)
  line L609 (2.9646, 27.9426) -> (3.0285, 27.7263)
  line L610 (3.0285, 27.7263) -> (3.085, 27.5195)
  line L611 (3.085, 27.5195) -> (3.1342, 27.3234)
  line L612 (3.1342, 27.3234) -> (3.1768, 27.1369)
  line L613 (3.1768, 27.1369) -> (3.2134, 26.9597)
  line L614 (3.2134, 26.9597) -> (3.2441, 26.7939)
  line L615 (3.2441, 26.7939) -> (3.2694, 26.6388)
  line L616 (3.2694, 26.6388) -> (3.3062, 26.3589)
  line L617 (3.3062, 26.3589) -> (3.3337, 26.0488)
  line L618 (3.3337, 26.0488) -> (3.3458, 25.9718)
  line L619 (3.3458, 25.9718) -> (3.3624, 25.9068)
  line L620 (3.3624, 25.9068) -> (3.383, 25.8539)
  line L621 (3.383, 25.8539) -> (3.4069, 25.8133)
  line L622 (3.4069, 25.8133) -> (3.4338, 25.7851)
  line L623 (3.4338, 25.7851) -> (3.4632, 25.7694)
  line L624 (3.4632, 25.7694) -> (3.4977, 25.7637)
  line L625 (3.4977, 25.7637) -> (3.7002, 25.7354)
  line L626 (3.7002, 25.7354) -> (3.9024, 25.7056)
  line L627 (3.9024, 25.7056) -> (3.9372, 25.7013)
  line L628 (3.9372, 25.7013) -> (3.9698, 25.7081)
  line L629 (3.9698, 25.7081) -> (4.0035, 25.7276)
  line L630 (4.0035, 25.7276) -> (4.038, 25.7598)
  line L631 (4.038, 25.7598) -> (4.0726, 25.8047)
  line L632 (4.0726, 25.8047) -> (4.1068, 25.8624)
  line L633 (4.1068, 25.8624) -> (4.1402, 25.9329)
  line L634 (4.1402, 25.9329) -> (4.2539, 26.2227)
  line L635 (4.2539, 26.2227) -> (4.368, 26.4808)
  line L636 (4.368, 26.4808) -> (4.4361, 26.6225)
  line L637 (4.4361, 26.6225) -> (4.5122, 26.773)
  line L638 (4.5122, 26.773) -> (4.5972, 26.9327)
  line L639 (4.5972, 26.9327) -> (4.6907, 27.0996)
  line L640 (4.6907, 27.0996) -> (4.7931, 27.2739)
  line L641 (4.7931, 27.2739) -> (4.9055, 27.4564)
  line L642 (4.9055, 27.4564) -> (5.0278, 27.6459)
  line L643 (5.0278, 27.6459) -> (5.1609, 27.8429)
  line L644 (5.1609, 27.8429) -> (5.2766, 28.0073)
  arc A16 (6.042, 27.8522) -> (5.2766, 28.0073) centre (0, 0) ccw
  line L645 (6.042, 27.8522) -> (6.0846, 27.6557)
  line L646 (6.0846, 27.6557) -> (6.1305, 27.4225)
  line L647 (6.1305, 27.4225) -> (6.1694, 27.2004)
  line L648 (6.1694, 27.2004) -> (6.2019, 26.9884)
  line L649 (6.2019, 26.9884) -> (6.2284, 26.788)
  line L650 (6.2284, 26.788) -> (6.2495, 26.5979)
  line L651 (6.2495, 26.5979) -> (6.2656, 26.4177)
  line L652 (6.2656, 26.4177) -> (6.2772, 26.2495)
  line L653 (6.2772, 26.2495) -> (6.2847, 26.0924)
  line L654 (6.2847, 26.0924) -> (6.2894, 25.8102)
  line L655 (6.2894, 25.8102) -> (6.2813, 25.499)
  line L656 (6.2813, 25.499) -> (6.2846, 25.4211)
  line L657 (6.2846, 25.4211) -> (6.2937, 25.3546)
  line L658 (6.2937, 25.3546) -> (6.308, 25.2998)
  line L659 (6.308, 25.2998) -> (6.3272, 25.2567)
  line L660 (6.3272, 25.2567) -> (6.3507, 25.2256)
  line L661 (6.3507, 25.2256) -> (6.3781, 25.2067)
  line L662 (6.3781, 25.2067) -> (6.4118, 25.1971)
  line L663 (6.4118, 25.1971) -> (6.6097, 25.1458)
  line L664 (6.6097, 25.1458) -> (6.8072, 25.0932)
  line L665 (6.8072, 25.0932) -> (6.8413, 25.085)
  line L666 (6.8413, 25.085) -> (6.8744, 25.088)
  line L667 (6.8744, 25.088) -> (6.9102, 25.1035)
  line L668 (6.9102, 25.1035) -> (6.948, 25.1316)
  line L669 (6.948, 25.1316) -> (6.9875, 25.1723)
  line L670 (6.9875, 25.1723) -> (7.0281, 25.2257)
  line L671 (7.0281, 25.2257) -> (7.0693, 25.2919)
  line L672 (7.0693, 25.2919) -> (7.2153, 25.5668)
  line L673 (7.2153, 25.5668) -> (7.3581, 25.8103)
  line L674 (7.3581, 25.8103) -> (7.4419, 25.9433)
  line L675 (7.4419, 25.9433) -> (7.5347, 26.0841)
  line L676 (7.5347, 26.0841) -> (7.6374, 26.2331)
  line L677 (7.6374, 26.2331) -> (7.7492, 26.3882)
  line L678 (7.7492, 26.3882) -> (7.8708, 26.5497)
  line L679 (7.8708, 26.5497) -> (8.0034, 26.7183)
  line L680 (8.0034, 26.7183) -> (8.1465, 26.8926)
  line L681 (8.1465, 26.8926) -> (8.3011, 27.0731)
  line L682 (8.3011, 27.0731) -> (8.4348, 27.2232)
  arc A17 (9.1775, 26.9819) -> (8.4348, 27.2232) centre (0, 0) ccw
  line L683 (9.1775, 26.9819) -> (9.1974, 26.7819)
  line L684 (9.1974, 26.7819) -> (9.2164, 26.5449)
  line L685 (9.2164, 26.5449) -> (9.2297, 26.3198)
  line L686 (9.2297, 26.3198) -> (9.2379, 26.1055)
  line L687 (9.2379, 26.1055) -> (9.2414, 25.9034)
  line L688 (9.2414, 25.9034) -> (9.2407, 25.7121)
  line L689 (9.2407, 25.7121) -> (9.2362, 25.5313)
  line L690 (9.2362, 25.5313) -> (9.2285, 25.3628)
  line L691 (9.2285, 25.3628) -> (9.218, 25.206)
  line L692 (9.218, 25.206) -> (9.1905, 24.925)
  line L693 (9.1905, 24.925) -> (9.147, 24.6168)
  line L694 (9.147, 24.6168) -> (9.1414, 24.539)
  line L695 (9.1414, 24.539) -> (9.1428, 24.472)
  line L696 (9.1428, 24.472) -> (9.1509, 24.4158)
  line L697 (9.1509, 24.4158) -> (9.165, 24.3708)
  line L698 (9.165, 24.3708) -> (9.1849, 24.3373)
  line L699 (9.1849, 24.3373) -> (9.2099, 24.3153)
  line L700 (9.2099, 24.3153) -> (9.2422, 24.302)
  line L701 (9.2422, 24.302) -> (9.433, 24.2285)
  line L702 (9.433, 24.2285) -> (9.6232, 24.1536)
  line L703 (9.6232, 24.1536) -> (9.6561, 24.1416)
  line L704 (9.6561, 24.1416) -> (9.6894, 24.1408)
  line L705 (9.6894, 24.1408) -> (9.7267, 24.1522)
  line L706 (9.7267, 24.1522) -> (9.7675, 24.1757)
  line L707 (9.7675, 24.1757) -> (9.8114, 24.2117)
  line L708 (9.8114, 24.2117) -> (9.8578, 24.2601)
  line L709 (9.8578, 24.2601) -> (9.9063, 24.3212)
  line L710 (9.9063, 24.3212) -> (10.0827, 24.5777)
  line L711 (10.0827, 24.5777) -> (10.2523, 24.8033)
  line L712 (10.2523, 24.8033) -> (10.3507, 24.9259)
  line L713 (10.3507, 24.9259) -> (10.4589, 25.0552)
  line L714 (10.4589, 25.0552) -> (10.5779, 25.1915)
  line L715 (10.5779, 25.1915) -> (10.7067, 25.3329)
  line L716 (10.7067, 25.3329) -> (10.846, 25.4795)
  line L717 (10.846, 25.4795) -> (10.9969, 25.6318)
  line L718 (10.9969, 25.6318) -> (11.1589, 25.7887)
  line L719 (11.1589, 25.7887) -> (11.3331, 25.9504)
  line L720 (11.3331, 25.9504) -> (11.4831, 26.0843)
  arc A18 (12.1934, 25.7599) -> (11.4831, 26.0843) centre (0, 0) ccw
  line L721 (12.1934, 25.7599) -> (12.1904, 25.5589)
  line L722 (12.1904, 25.5589) -> (12.1823, 25.3213)
  line L723 (12.1823, 25.3213) -> (12.1698, 25.0961)
  line L724 (12.1698, 25.0961) -> (12.1535, 24.8823)
  line L725 (12.1535, 24.8823) -> (12.1339, 24.6811)
  line L726 (12.1339, 24.6811) -> (12.1114, 24.4912)
  line L727 (12.1114, 24.4912) -> (12.0863, 24.312)
  line L728 (12.0863, 24.312) -> (12.0595, 24.1455)
  line L729 (12.0595, 24.1455) -> (12.0312, 23.9909)
  line L730 (12.0312, 23.9909) -> (11.9718, 23.7149)
  line L731 (11.9718, 23.7149) -> (11.8935, 23.4137)
  line L732 (11.8935, 23.4137) -> (11.8791, 23.337)
  line L733 (11.8791, 23.337) -> (11.8728, 23.2702)
  line L734 (11.8728, 23.2702) -> (11.8744, 23.2135)
  line L735 (11.8744, 23.2135) -> (11.8834, 23.1673)
  line L736 (11.8834, 23.1673) -> (11.8992, 23.1317)
  line L737 (11.8992, 23.1317) -> (11.9216, 23.107)
  line L738 (11.9216, 23.107) -> (11.9522, 23.09)
  line L739 (11.9522, 23.09) -> (12.1334, 22.9953)
  line L740 (12.1334, 22.9953) -> (12.3138, 22.8992)
  line L741 (12.3138, 22.8992) -> (12.3451, 22.8835)
  line L742 (12.3451, 22.8835) -> (12.3781, 22.879)
  line L743 (12.3781, 22.879) -> (12.4164, 22.886)
  line L744 (12.4164, 22.886) -> (12.4597, 22.9047)
  line L745 (12.4597, 22.9047) -> (12.5074, 22.9354)
  line L746 (12.5074, 22.9354) -> (12.559, 22.9783)
  line L747 (12.559, 22.9783) -> (12.6141, 23.0334)
  line L748 (12.6141, 23.0334) -> (12.8186, 23.2682)
  line L749 (12.8186, 23.2682) -> (13.0129, 23.4729)
  line L750 (13.0129, 23.4729) -> (13.1246, 23.5835)
  line L751 (13.1246, 23.5835) -> (13.2468, 23.6997)
  line L752 (13.2468, 23.6997) -> (13.3806, 23.8215)
  line L753 (13.3806, 23.8215) -> (13.5247, 23.9473)
  line L754 (13.5247, 23.9473) -> (13.6797, 24.077)
  line L755 (13.6797, 24.077) -> (13.847, 24.2112)
  line L756 (13.847, 24.2112) -> (14.0258, 24.3485)
  line L757 (14.0258, 24.3485) -> (14.2173, 24.4894)
  line L758 (14.2173, 24.4894) -> (14.3816, 24.6053)
  arc A19 (15.0503, 24.202) -> (14.3816, 24.6053) centre (0, 0) ccw
  line L759 (15.0503, 24.202) -> (15.0244, 24.0027)
  line L760 (15.0244, 24.0027) -> (14.9893, 23.7676)
  line L761 (14.9893, 23.7676) -> (14.9512, 23.5453)
  line L762 (14.9512, 23.5453) -> (14.9106, 23.3347)
  line L763 (14.9106, 23.3347) -> (14.8682, 23.1371)
  line L764 (14.8682, 23.1371) -> (14.8242, 22.9509)
  line L765 (14.8242, 22.9509) -> (14.7789, 22.7758)
  line L766 (14.7789, 22.7758) -> (14.7333, 22.6135)
  line L767 (14.7333, 22.6135) -> (14.6875, 22.463)
  line L768 (14.6875, 22.463) -> (14.5971, 22.1957)
  line L769 (14.5971, 22.1957) -> (14.4849, 21.9053)
  line L770 (14.4849, 21.9053) -> (14.4618, 21.8308)
  line L771 (14.4618, 21.8308) -> (14.4481, 21.7652)
  line L772 (14.4481, 21.7652) -> (14.4432, 21.7086)
  line L773 (14.4432, 21.7086) -> (14.4468, 21.6616)
  line L774 (14.4468, 21.6616) -> (14.4585, 21.6245)
  line L775 (14.4585, 21.6245) -> (14.4779, 21.5974)
  line L776 (14.4779, 21.5974) -> (14.5064, 21.5771)
  line L777 (14.5064, 21.5771) -> (14.6755, 21.4623)
  line L778 (14.6755, 21.4623) -> (14.8439, 21.3463)
  line L779 (14.8439, 21.3463) -> (14.8732, 21.3271)
  line L780 (14.8732, 21.3271) -> (14.9054, 21.3189)
  line L781 (14.9054, 21.3189) -> (14.9443, 21.3214)
  line L782 (14.9443, 21.3214) -> (14.9894, 21.3351)
  line L783 (14.9894, 21.3351) -> (15.0403, 21.3602)
  line L784 (15.0403, 21.3602) -> (15.0965, 21.3969)
  line L785 (15.0965, 21.3969) -> (15.1575, 21.4454)
  line L786 (15.1575, 21.4454) -> (15.3874, 21.6553)
  line L787 (15.3874, 21.6553) -> (15.6038, 21.8366)
  line L788 (15.6038, 21.8366) -> (15.7273, 21.9337)
  line L789 (15.7273, 21.9337) -> (15.862, 22.0352)
  line L790 (15.862, 22.0352) -> (16.0088, 22.1409)
  line L791 (16.0088, 22.1409) -> (16.1663, 22.2495)
  line L792 (16.1663, 22.2495) -> (16.3351, 22.3607)
  line L793 (16.3351, 22.3607) -> (16.5166, 22.4749)
  line L794 (16.5166, 22.4749) -> (16.7099, 22.591)
  line L795 (16.7099, 22.591) -> (16.9163, 22.7091)
  line L796 (16.9163, 22.7091) -> (17.0926, 22.8055)
  arc A20 (17.711, 22.3287) -> (17.0926, 22.8055) centre (0, 0) ccw
  line L797 (17.711, 22.3287) -> (17.6626, 22.1336)
  line L798 (17.6626, 22.1336) -> (17.6009, 21.904)
  line L799 (17.6009, 21.904) -> (17.5377, 21.6875)
  line L800 (17.5377, 21.6875) -> (17.4734, 21.483)
  line L801 (17.4734, 21.483) -> (17.4088, 21.2914)
  line L802 (17.4088, 21.2914) -> (17.3438, 21.1115)
  line L803 (17.3438, 21.1115) -> (17.2788, 20.9427)
  line L804 (17.2788, 20.9427) -> (17.215, 20.7866)
  line L805 (17.215, 20.7866) -> (17.1524, 20.6424)
  line L806 (17.1524, 20.6424) -> (17.0321, 20.387)
  line L807 (17.0321, 20.387) -> (16.8875, 20.1113)
  line L808 (16.8875, 20.1113) -> (16.8561, 20.04)
  line L809 (16.8561, 20.04) -> (16.8349, 19.9763)
  line L810 (16.8349, 19.9763) -> (16.8236, 19.9208)
  line L811 (16.8236, 19.9208) -> (16.8218, 19.8736)
  line L812 (16.8218, 19.8736) -> (16.8292, 19.8354)
  line L813 (16.8292, 19.8354) -> (16.8454, 19.8063)
  line L814 (16.8454, 19.8063) -> (16.8714, 19.7828)
  line L815 (16.8714, 19.7828) -> (17.0264, 19.6495)
  line L816 (17.0264, 19.6495) -> (17.1804, 19.5151)
  line L817 (17.1804, 19.5151) -> (17.2073, 19.4927)
  line L818 (17.2073, 19.4927) -> (17.2384, 19.4808)
  line L819 (17.2384, 19.4808) -> (17.2774, 19.4789)
  line L820 (17.2774, 19.4789) -> (17.3237, 19.4874)
  line L821 (17.3237, 19.4874) -> (17.3771, 19.5065)
  line L822 (17.3771, 19.5065) -> (17.4371, 19.5365)
  line L823 (17.4371, 19.5365) -> (17.5033, 19.5778)
  line L824 (17.5033, 19.5778) -> (17.7556, 19.7601)
  line L825 (17.7556, 19.7601) -> (17.9912, 19.9155)
  line L826 (17.9912, 19.9155) -> (18.1251, 19.998)
  line L827 (18.1251, 19.998) -> (18.2705, 20.0834)
  line L828 (18.2705, 20.0834) -> (18.4283, 20.1717)
  line L829 (18.4283, 20.1717) -> (18.5972, 20.2616)
  line L830 (18.5972, 20.2616) -> (18.7776, 20.3529)
  line L831 (18.7776, 20.3529) -> (18.9709, 20.4457)
  line L832 (18.9709, 20.4457) -> (19.1762, 20.539)
  line L833 (19.1762, 20.539) -> (19.3946, 20.6327)
  line L834 (19.3946, 20.6327) -> (19.5809, 20.7085)
  arc A21 (20.1409, 20.1642) -> (19.5809, 20.7085) centre (0, 0) ccw
  line L835 (20.1409, 20.1642) -> (20.0705, 19.9759)
  line L836 (20.0705, 19.9759) -> (19.983, 19.7549)
  line L837 (19.983, 19.7549) -> (19.8956, 19.547)
  line L838 (19.8956, 19.547) -> (19.8084, 19.3511)
  line L839 (19.8084, 19.3511) -> (19.7223, 19.1682)
  line L840 (19.7223, 19.1682) -> (19.6373, 18.9968)
  line L841 (19.6373, 18.9968) -> (19.5535, 18.8365)
  line L842 (19.5535, 18.8365) -> (19.4722, 18.6887)
  line L843 (19.4722, 18.6887) -> (19.3937, 18.5526)
  line L844 (19.3937, 18.5526) -> (19.245, 18.3126)
  line L845 (19.245, 18.3126) -> (19.07, 18.0552)
  line L846 (19.07, 18.0552) -> (19.0306, 17.9879)
  line L847 (19.0306, 17.9879) -> (19.0023, 17.9271)
  line L848 (19.0023, 17.9271) -> (18.9847, 17.8732)
  line L849 (18.9847, 17.8732) -> (18.9776, 17.8266)
  line L850 (18.9776, 17.8266) -> (18.9806, 17.7877)
  line L851 (18.9806, 17.7877) -> (18.9934, 17.757)
  line L852 (18.9934, 17.757) -> (19.0165, 17.7307)
  line L853 (19.0165, 17.7307) -> (19.1553, 17.5805)
  line L854 (19.1553, 17.5805) -> (19.293, 17.4295)
  line L855 (19.293, 17.4295) -> (19.3172, 17.4041)
  line L856 (19.3172, 17.4041) -> (19.3467, 17.3888)
  line L857 (19.3467, 17.3888) -> (19.3852, 17.3825)
  line L858 (19.3852, 17.3825) -> (19.4322, 17.3856)
  line L859 (19.4322, 17.3856) -> (19.4874, 17.3985)
  line L860 (19.4874, 17.3985) -> (19.5505, 17.4215)
  line L861 (19.5505, 17.4215) -> (19.6209, 17.4549)
  line L862 (19.6209, 17.4549) -> (19.8924, 17.6073)
  line L863 (19.8924, 17.6073) -> (20.1442, 17.7349)
  line L864 (20.1442, 17.7349) -> (20.2865, 17.8015)
  line L865 (20.2865, 17.8015) -> (20.4407, 17.8698)
  line L866 (20.4407, 17.8698) -> (20.6076, 17.9396)
  line L867 (20.6076, 17.9396) -> (20.7856, 18.0097)
  line L868 (20.7856, 18.0097) -> (20.9752, 18.0798)
  line L869 (20.9752, 18.0798) -> (21.1779, 18.1499)
  line L870 (21.1779, 18.1499) -> (21.3925, 18.2192)
  line L871 (21.3925, 18.2192) -> (21.6202, 18.2874)
  line L872 (21.6202, 18.2874) -> (21.8138, 18.3414)
  arc A22 (22.3081, 17.7369) -> (21.8138, 18.3414) centre (0, 0) ccw
  line L873 (22.3081, 17.7369) -> (22.2167, 17.5578)
  line L874 (22.2167, 17.5578) -> (22.1046, 17.3482)
  line L875 (22.1046, 17.3482) -> (21.9941, 17.1517)
  line L876 (21.9941, 17.1517) -> (21.8851, 16.967)
  line L877 (21.8851, 16.967) -> (21.7788, 16.7951)
  line L878 (21.7788, 16.7951) -> (21.6748, 16.6345)
  line L879 (21.6748, 16.6345) -> (21.5732, 16.4848)
  line L880 (21.5732, 16.4848) -> (21.4757, 16.3473)
  line L881 (21.4757, 16.3473) -> (21.3821, 16.221)
  line L882 (21.3821, 16.221) -> (21.207, 15.9995)
  line L883 (21.207, 15.9995) -> (21.0038, 15.7637)
  line L884 (21.0038, 15.7637) -> (20.957, 15.7013)
  line L885 (20.957, 15.7013) -> (20.922, 15.6441)
  line L886 (20.922, 15.6441) -> (20.8984, 15.5926)
  line L887 (20.8984, 15.5926) -> (20.886, 15.5471)
  line L888 (20.886, 15.5471) -> (20.8845, 15.5081)
  line L889 (20.8845, 15.5081) -> (20.8937, 15.4761)
  line L890 (20.8937, 15.4761) -> (20.9137, 15.4474)
  line L891 (20.9137, 15.4474) -> (21.0344, 15.2824)
  line L892 (21.0344, 15.2824) -> (21.154, 15.1166)
  line L893 (21.154, 15.1166) -> (21.1752, 15.0887)
  line L894 (21.1752, 15.0887) -> (21.2028, 15.0701)
  line L895 (21.2028, 15.0701) -> (21.2403, 15.0594)
  line L896 (21.2403, 15.0594) -> (21.2874, 15.0572)
  line L897 (21.2874, 15.0572) -> (21.3437, 15.0637)
  line L898 (21.3437, 15.0637) -> (21.4089, 15.0794)
  line L899 (21.4089, 15.0794) -> (21.4827, 15.1045)
  line L900 (21.4827, 15.1045) -> (21.7698, 15.225)
  line L901 (21.7698, 15.225) -> (22.0345, 15.323)
  line L902 (22.0345, 15.323) -> (22.1835, 15.373)
  line L903 (22.1835, 15.373) -> (22.3445, 15.4233)